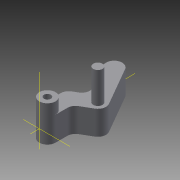
# Autodesk Inventor part: arm
Saved by Autodesk Inventor 2014 (Build 180170000, 170)
## iProperties
Created: 2014-11-20
Part Number: arm
Material: Generic
Document SubType Name: Modeling
Designer: KriMag
Density: 1 g/cm^3
Appearance: Default
Author: KriMag
Autodesk Inventor part; units mm, degrees
ref_plane "YZ Plane" through (0, 0, 0) normal (1, 0, 0) x (0, 1, 0)
ref_plane "XZ Plane" through (0, 0, 0) normal (0, 1, 0) x (-1, 0, 0)
ref_plane "XY Plane" through (0, 0, 0) normal (0, 0, 1) x (1, 0, 0)
sketch "Sketch2" plane through (0, 0, 0) normal (0, 1, 0) x (-1, 0, 0)
  line L0 (3.5, -5.25) -> (-3.5, -5.25)
  line L1 (-3.5, -5.25) -> (-3.5, 5.25)
  line L2 (-3.5, 5.25) -> (3.5, 5.25)
  line L3 (3.5, 5.25) -> (3.5, -5.25)
  line L4 (3.5, -5.25) -> (-3.5, 5.25) construction
  line L5 (-3.5, -5.25) -> (3.5, 5.25) construction
  point P0 (0, 0)
  dimension "d11" = 10.5
  dimension "d12" = 7
  constraints: 12 end point, 2 midpoint, 2 parallel, 1 horizontal, 1 perpendicular
  measures "d11" distance of L0.end L1.end
  measures "d12" distance of L1.end L2.end
sketch "Sketch3" plane through (0, 0, 0) normal (0, 0, 1) x (1, 0, 0)
  line L0 (0, 0) -> (0, 12.75)
  line L1 (0, 12.75) -> (8.0107, 17.375)
  line L2 (8.0107, 17.375) -> (-3.3643, 37.0771)
  dimension "d13" = 12.75
  dimension "d14" = 9.25
  dimension "d15" = 120
  dimension "d16" = 22.75
  dimension "d30" = 90
  constraints: 6 end point, 1 vertical
  measures "d13" distance of L0.start L0.end
  measures "d14" distance of L0.end L1.end
  measures "d15" angle of L0 L1
  measures "d16" distance of L1.end L2.end
  measures "d30" angle of L1 L2
sweep "Sweep1" add profiles "Sketch2" path "Sketch3"
sketch "Sketch4" plane through (-3.5, 0, 5.25) normal (0, 0, 1) x (1, 0, 0)
  line L0 (7, 0) -> (0, 0) projected
  circle A0 centre (3.5, 3.5) radius 1.5
  point P0 (3.5, 0)
  point P1 (3.5, 0)
  dimension "d19" = 3
  dimension "d20" = 3.5
  constraints: 1 centre point, 1 midpoint, 1 vertical alignment
  measures "d19" diameter of A0
  measures "d20" distance from line of A0.centre L0
extrude "Extrusion1" cut sketch "Sketch4" against normal blind 11.5
sketch "Sketch5" plane through (-3.5, 0, 5.25) normal (0, 0, 1) x (1, 0, 0)
  line L0 (6.7296, 18.6561) -> (16.2918, 16.0939) construction
  circle A0 centre (11.5107, 17.375) radius 2
  point P0 (3.5, 0)
  dimension "d24" = 4
  constraints: 2 end point, 1 centre point, 1 midpoint
  measures "d24" diameter of A0
extrude "Extrusion2" add sketch "Sketch5" along normal blind 13.5
fillet "Fillet2" radius 3.5 8 edges at (3.5, 0, 0) (-3.5, 0, 0) (3.5, 10.7293, 0) (-0.3332, 38.8271, 0) (12.7918, 16.0939, 0) (-3.5, 14.7707, 0) (3.2296, 18.6561, 0) (-6.3954, 35.3271, 0)
sketch "Sketch6" plane through (-1.6143, 34.046, 5.25) normal (0, 0, 1) x (0.8660254, 0.5, 0)
  circle A0 centre (-13.875, -27.2607) radius 1.5 projected
  arc A1 (-16.9061, -25.5107) -> (-10.8439, -29.0107) centre (-13.875, -27.2607) ccw projected
  circle A2 centre (-13.875, -27.2607) radius 3.5
  point P0 (-15.625, -30.2918)
  constraints: 1 coincident, 3 other
extrude "Extrusion3" add sketch "Sketch6" along normal blind 5
body "Solid1"
